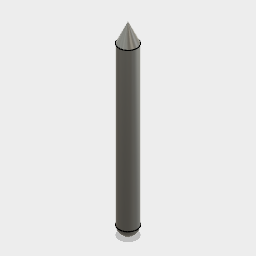
pencil (Autodesk Fusion 360 design; units mm, degrees)
Autodesk Fusion 360 part; units mm, degrees
cylinder "圆柱体基本要素1" add diameter 10 height 75 placed x (1, 0, 0) y (0, 0, -1) z (0, 1, 0) at (0, 0, 0) makes body 1
sphere "球体基本要素1" add diameter 10 placed x (1, 0, 0) y (0, 0, -1) z (0, 1, 0) at (10, 0, 10) separate body makes body 2
move_body "MoveFace1" bodies 2 to x (1, 0, 0) y (0, 1, 0) z (0, 0, 1) at (-2.6751, 5.7664, -3.0913) on bodies 2
move_body "MoveFace2" bodies 2 to x (1, 0, 0) y (0, 1, 0) z (0, 0, 1) at (-9.126, -5.4654, -4.3471) on bodies 2
move_body "MoveFace3" bodies 2 to x (1, 0, 0) y (0, 1, 0) z (0, 0, 1) at (2.3304, -0.0333, -1.8904) on bodies 2
move_body "MoveFace4" bodies 2 to x (1, 0, 0) y (0, 1, 0) z (0, 0, 1) at (-0.8937, 1.1765, -0.5729) on bodies 2
delete_face "删除面1" 1 faces at (4.3759, 2.6261, -0.9656) on bodies 2
sphere "球体基本要素2" cut diameter 10 placed x (1, 0, 0) y (0, 0, 1) z (0, -1, 0) at (0, 0, 0) bodies 1
sphere "球体基本要素3" add diameter 10 placed x (1, 0, 0) y (0, 0, -1) z (0, 1, 0) at (0, 0, 0) bodies 1
move_face "偏移面1" offset 13 1 faces at (1.3101, 75, 1.9935) on bodies 1
extrude "拉伸1" add 1 faces at (1.3101, 88, 1.9935) along direction (0, 1, 0) blind 25 draft -25 on bodies 1 bodies 1
